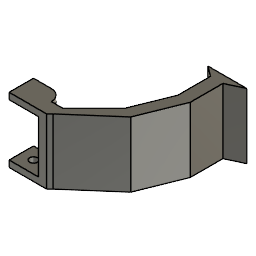
neck (Assembly) (Autodesk Fusion 360 archive; units mm, degrees)
design "tib 1"
Autodesk Fusion 360 part; units mm, degrees
note: some values were not read from the file. Chosen so that the rebuilt part matches the saved one: which face or edge a step refers to; which pieces of a blend or face edit are solid. Set by a fixed rule: which sketch regions a step uses.
sketch "Sketch1" plane through (0, 0, 0) normal (0, 0, 1) x (1, 0, 0)
  line L0 (0, 0) -> (50, 0)
  line L1 (50, 0) -> (50, 15)
  line L2 (50, 15) -> (0, 15)
  line L3 (0, 15) -> (0, 0)
  constraint horizontal L0
  constraint vertical L1
  constraint horizontal L2
  constraint vertical L3
  constraint coincident L0.start L3.end
extrude "Extrude1" add sketch "Sketch1" along normal blind 40
sketch "Sketch2" plane through (0, 0, 0) normal (-1, 0, 0) x (0, -1, 0)
  line L0 (-15, 0) -> (0, 0)
  line L1 (0, 0) -> (0, 40)
  line L2 (0, 40) -> (-15, 40)
  line L3 (-15, 40) -> (-15, 0)
  line L4 (2.957876, 2) -> (-22.207484, 2)
  line L5 (-22.207484, 2) -> (-22.207484, 38.000001)
  line L6 (-22.207484, 38.000001) -> (2.957876, 38.000001)
  line L7 (2.957876, 38.000001) -> (2.957876, 2)
  constraint horizontal L4
  constraint vertical L5
  constraint horizontal L6
  constraint vertical L7
extrude "Extrude2" cut sketch "Sketch2" against normal blind 46 contours L1 L3 L4 L6 picked at (-10, 26)
sketch "Sketch3" plane through (0, 0, 40) normal (0, 0, 1) x (-1, 0, 0)
  line L0 (0, -15) -> (0, 0)
  line L1 (0, 0) -> (-50, 0)
  line L2 (-50, 0) -> (-50, -15)
  line L3 (-50, -15) -> (0, -15)
  circle A0 centre (-7.5, -7.5) radius 2.4
  dimension "d5" = 4.8
  measures "d5" diameter of A0
extrude "Extrude3" cut sketch "Sketch3" against normal blind 50 contours A0 picked at (-7.452057, -6.860244)
sketch "Sketch4" plane through (0, 0, 0) normal (0, 0, -1) x (1, 0, 0)
  circle A0 centre (7.5, -7.5) radius 2.4
  line L0 (0, 0) -> (0, -15)
  line L1 (0, -15) -> (50, -15)
  line L2 (50, -15) -> (50, 0)
  line L3 (50, 0) -> (0, 0)
  circle A1 centre (7.5, -7.5) radius 4
  dimension "d8" = 8
  constraint concentric A0 A1
  measures "d8" diameter of A1
extrude "Extrude4" cut sketch "Sketch4" against normal blind 7 contours A1 picked at (10.951775, -7.698723)
extrude "Extrude5" add 1 faces at (46, 10, 26) along direction (-1, 0, 0) blind 30
extrude "Extrude6" cut 1 faces at (50, 5, 26.666667) along direction (-1, 0, 0) blind 25
chamfer "Chamfer1" distance 7 angle 45 1 edges at (25, 15, 20)
chamfer "Chamfer2" distance 2 angle 45 1 edges at (25, 0, 20)
extrude "Extrude7" add 1 faces at (22.666667, 10.333333, 13.333333) along direction (0.70710678, 0.70710678, 0) blind 30
chamfer "Chamfer3" distance 7 angle 45 1 edges at (39.213203, 36.213203, 20)
extrude "Extrude8" add 1 faces at (40.863119, 31.263456, 13.333333) along direction (0, 1, 0) blind 25
sketch "Sketch5" plane through (0, 0, 0) normal (0, 0, -1) x (1, 0, 0)
  circle A0 centre (7.5, -7.5) radius 4
  line L0 (44.162951, -31.263456) -> (46.213203, -29.213203)
  line L1 (46.213203, -29.213203) -> (25, -8)
  line L2 (25, -8) -> (25, -2)
  line L3 (25, -2) -> (23, 0)
  line L4 (23, 0) -> (0, 0)
  line L5 (0, 0) -> (0, -15)
  line L6 (0, -15) -> (18, -15)
  line L7 (18, -15) -> (34.263456, -31.263456)
  line L8 (34.263456, -31.263456) -> (34.263456, -56.263456)
  line L9 (34.263456, -56.263456) -> (44.162951, -56.263456)
  line L10 (44.162951, -56.263456) -> (44.162951, -31.263456)
  line L11 (44.162951, -31.263456) -> (44.162951, -27.162951)
  line L12 (44.162951, -27.162951) -> (46.213203, -29.213203)
  line L13 (44.162951, -31.263456) -> (46.213203, -29.213203)
  constraint parallel L10 L11
extrude "Extrude9" cut sketch "Sketch5" against normal blind 43 contours L0 L1 L11 L12 L13 picked at (44.846368, -29.213203)
chamfer "Chamfer4" distance 3 angle 45 1 edges at (44.162951, 56.263456, 20)
sketch "Sketch6" plane through (0, 0, 0) normal (0, 0, -1) x (1, 0, 0)
  line L0 (41.162951, -56.263456) -> (44.162951, -53.263456)
  line L1 (44.162951, -53.263456) -> (44.162951, -27.162951)
  line L2 (44.162951, -27.162951) -> (25, -8)
  line L3 (25, -8) -> (25, -2)
  line L4 (25, -2) -> (23, 0)
  line L5 (23, 0) -> (0, 0)
  line L6 (0, 0) -> (0, -15)
  line L7 (0, -15) -> (18, -15)
  line L8 (18, -15) -> (34.263456, -31.263456)
  line L9 (34.263456, -31.263456) -> (34.263456, -56.263456)
  line L10 (34.263456, -56.263456) -> (41.162951, -56.263456)
  circle A0 centre (7.5, -7.5) radius 4
  circle A1 centre (7.5, -7.5) radius 2.4
  dimension "d25" = 4.8
  constraint concentric A0 A1
  measures "d25" diameter of A1
extrude "Extrude10" add sketch "Sketch6" against normal blind 2 contours A0 picked at (10.951775, -7.698723)
sketch "Sketch7" plane through (0, 0, 38.000001) normal (0, 0, -1) x (1, 0, 0)
  line L0 (16, -15) -> (16, 0)
  line L1 (16, 0) -> (0, 0)
  line L2 (0, 0) -> (0, -15)
  line L3 (0, -15) -> (16, -15)
  circle A0 centre (7.5, -7.5) radius 2.4
  circle A1 centre (7.5, -7.5) radius 4
  dimension "d28" = 8
  constraint concentric A0 A1
  measures "d28" diameter of A1
extrude "Extrude11" cut sketch "Sketch7" against normal blind 3 contours A1 picked at (10.951775, -7.698723)
sketch "Sketch8" plane through (0, 0, 38.000001) normal (0, 0, -1) x (1, 0, 0)
  circle A0 centre (7.5, -7.5) radius 4
  line L0 (16, -15) -> (16, 0)
  line L1 (16, 0) -> (0, 0)
  line L2 (0, 0) -> (0, -15)
  line L3 (0, -15) -> (16, -15)
  circle A1 centre (7.5, -7.5) radius 4
  constraint concentric A0 A1
extrude "Extrude12" add sketch "Sketch8" along normal blind 2 and the other way blind 2 contours A0 A1 picked at (6.101654, -8.048811)
extrude "Extrude13" cut 1 faces at (36.563288, 56.263456, 26.666667) along direction (0, -1, 0) blind 25
sketch "Sketch9" plane through (0, 0, 40) normal (0, 0, 1) x (-1, 0, 0)
  line L0 (-41.162951, -56.263456) -> (-41.162951, -31.263456)
  line L1 (-41.162951, -31.263456) -> (-34.263456, -31.263456)
  line L2 (-34.263456, -31.263456) -> (-18, -15)
  line L3 (-18, -15) -> (0, -15)
  line L4 (0, -15) -> (0, 0)
  line L5 (0, 0) -> (-23, 0)
  line L6 (-23, 0) -> (-25, -2)
  line L7 (-25, -2) -> (-25, -8)
  line L8 (-25, -8) -> (-44.162951, -27.162951)
  line L9 (-44.162951, -27.162951) -> (-44.162951, -53.263456)
  line L10 (-44.162951, -53.263456) -> (-41.162951, -56.263456)
extrude "Extrude14" cut 1 faces at (41.162951, 47.930123, 13.333333) along direction (1, 0, 0) blind 26
sketch "Sketch10" plane through (0, 0, 40) normal (0, 0, 1) x (-1, 0, 0)
  line L0 (-44.000001, -27) -> (-34.000001, -31)
  line L1 (-34.000001, -31) -> (-34.243008, -31.24155)
  line L2 (-34.243008, -31.24155) -> (-44.199999, -31.24155)
  line L3 (-44.199999, -31.24155) -> (-44.199999, -27.099999)
  line L4 (-44.199999, -27.099999) -> (-44.000001, -27)
  constraint horizontal L2
  constraint perpendicular L2 L3
extrude "Extrude15" cut sketch "Sketch10" against normal blind 45
delete_face "DeleteFace1" 1 faces at (40.863119, 31.263456, 13.333333)
delete_face "DeleteFace2" 1 faces at (40.856303, 34.548684, 40)
extrude "Extrude16" add 2 faces at (40.666667, 28.333334, 36.161338) (40.666667, 28.333334, 18.989342) along direction (0.37139068, 0.92847669, 0) blind 40
chamfer "Chamfer5" distance 5 angle 45 1 edges at (58.855628, 64.139068, 20)
extrude "Extrude17" add 1 faces at (13.966667, 7.5, 2) along direction (0, 0, 1) blind 4
extrude "Extrude18" cut 1 faces at (46.618101, 52.878584, 0) along direction (0, 0, 1) blind 2
extrude "Extrude19" cut 1 faces at (16, 10, 16.666667) along direction (1, 0, 0) blind 2
sketch "Sketch11" plane through (0, 0, 40) normal (0, 0, 1) x (-1, 0, 0)
  line L0 (-56.998674, -59.496685) -> (-54.213244, -65.996021)
  line L1 (-54.213244, -65.996021) -> (-48.855628, -68.139068)
  line L2 (-48.855628, -68.139068) -> (-34.000001, -31)
  line L3 (-34.000001, -31) -> (-18, -15)
  line L4 (-18, -15) -> (0, -15)
  line L5 (0, -15) -> (0, 0)
  line L6 (0, 0) -> (-23, 0)
  line L7 (-23, 0) -> (-25, -2)
  line L8 (-25, -2) -> (-25, -8)
  line L9 (-25, -8) -> (-44.000001, -27)
  line L10 (-44.000001, -27) -> (-56.998674, -59.496685)
  line L11 (-56.998674, -59.496685) -> (-60.937867, -50.305234)
  line L12 (-60.937867, -50.305234) -> (-50.499337, -24.208909)
  line L13 (-50.499337, -24.208909) -> (-25, -2)
  line L14 (-18, -15) -> (-18, -8)
  line L15 (-18, -8) -> (-25, -8)
  dimension "d50" = 10
  constraint parallel L0 L11
  constraint parallel L10 L12
  constraint coincident L7.end L8.start
  constraint coincident L3.end L4.start
  constraint perpendicular L4 L14
  constraint coincident L8.end L9.start
extrude "Extrude20" add sketch "Sketch11" against normal blind 38 contours L8 L9 L10 L11 L12 L13 picked at (-53.978847, -45.60064)
extrude "Extrude21" cut sketch "Sketch11" against normal blind 40 contours L0 L1 L2 L3 L9 L10 L14 L15 picked at (-46.618101, -52.878584)
extrude "Extrude22" add sketch "Sketch11" along normal blind 2 contours L8 L9 L10 L11 L12 L13 | L4 L5 L6 L7 L8 L14 L15 picked at (-53.978847, -45.60064) picked at (-6, -7.666667)
fillet "Fillet1" radius 7 2 edges at (18, 15, 4) (18, 15, 40)
sketch "Sketch15" plane through (0, 0, 42) normal (0, 0, 1) x (-1, 0, 0)
  arc A0 (-18, -8) -> (-11, -15) centre (-11, -8) ccw
  line L0 (-11, -15) -> (0, -15)
  line L1 (0, -15) -> (0, 0)
  line L2 (0, 0) -> (-23, 0)
  line L3 (-23, 0) -> (-25, -2)
  line L4 (-25, -2) -> (-50.499337, -24.208909)
  line L5 (-50.499337, -24.208909) -> (-60.937867, -50.305234)
  line L6 (-60.937867, -50.305234) -> (-56.998674, -59.496685)
  line L7 (-56.998674, -59.496685) -> (-44.000001, -27)
  line L8 (-44.000001, -27) -> (-25, -8)
  line L9 (-25, -8) -> (-18, -8)
  line L10 (-60.937867, -50.305234) -> (-53.322094, -50.305234)
  line L11 (-53.322094, -50.305234) -> (-56.998674, -59.496685)
  line L12 (-61.161175, -50.305234) -> (-56.998674, -59.496685)
  line L13 (-61.161175, -50.305234) -> (-60.899999, -50.305234)
  constraint horizontal L10
  constraint parallel L10 L13
extrude "Extrude23" cut sketch "Sketch15" against normal blind 41 contours L6 L7 L10 L11 L13 picked at (-57.073589, -53.369051)
extrude "Extrude24" add 1 faces at (58.399276, 50.305234, 28.666667) along direction (0, 1, 0) blind 20
sketch "Sketch16" plane through (0, 0, 2) normal (0, 0, -1) x (1, 0, 0)
  circle A0 centre (7.5, -7.5) radius 2.4
  line L0 (60.937867, -50.305234) -> (50.499337, -24.208909)
  line L1 (50.499337, -24.208909) -> (25, -2)
  line L2 (25, -2) -> (23, 0)
  line L3 (23, 0) -> (0, 0)
  line L4 (0, 0) -> (0, -15)
  line L5 (0, -15) -> (11, -15)
  arc A1 (11, -15) -> (18, -8) centre (11, -8) ccw
  line L6 (18, -8) -> (25, -8)
  line L7 (25, -8) -> (44.000001, -27)
  line L8 (44.000001, -27) -> (53.322094, -50.305234)
  line L9 (53.322094, -50.305234) -> (53.322094, -70.305234)
  line L10 (53.322094, -70.305234) -> (60.937867, -70.305234)
  line L11 (60.937867, -70.305234) -> (60.937867, -50.305234)
  line L12 (71.000001, -75.000001) -> (60.937867, -70.305234)
  line L13 (53.322094, -70.305234) -> (47.000001, -75.000001)
  line L14 (47.000001, -75.000001) -> (71.000001, -75.000001)
  constraint perpendicular L9 L14
extrude "Extrude25" add sketch "Sketch16" against normal blind 40 contours L10 L12 L13 L14 picked at (59.645956, -73.435079)

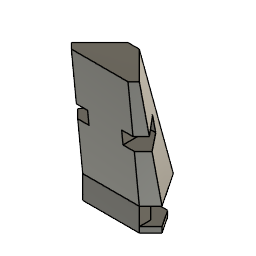
design "neck"
Autodesk Fusion 360 part; units mm, degrees
sketch "Sketch1" plane through (0, 0, 0) normal (0, 0, 1) x (1, 0, 0)
  line L0 (50, 30) -> (20, 30)
  line L1 (0, 0) -> (20, 30)
  line L2 (50, 30) -> (70, 0)
  line L3 (0, 0) -> (10, -10)
  line L4 (10, -10) -> (60, -10)
  line L5 (60, -10) -> (70, 0)
  constraint horizontal L0
  constraint coincident L1.start L3.start
  constraint perpendicular L3 L5
ref_plane "WorkPlane1" through (0, 0, 100) normal (0, 0, 1) x (1, 0, 0)
sketch "Sketch2" plane through (0, 0, 100) normal (0, 0, 1) x (1, 0, 0)
  line L0 (30, 10) -> (40, 10)
  line L1 (60, -20) -> (10, -20)
  line L2 (30, 10) -> (5, -15)
  line L3 (5, -15) -> (10, -20)
  line L4 (40, 10) -> (65, -15)
  line L5 (65, -15) -> (60, -20)
  constraint horizontal L0
  constraint horizontal L1
  constraint perpendicular L2 L3
  constraint parallel L3 L4
  constraint perpendicular L4 L5
loft "Loft1" add profiles "Sketch1", "Sketch2" section 1 section 2 makes body 1
ref_plane "WorkPlane2" through (35, 10, 50) normal (0, 0, -1) x (-1, 0, 0)
sketch "Sketch3" plane through (0, 0, 50) normal (0, 0, -1) x (-1, 0, 0)
  line L0 (0.4452, 9.35) -> (-20, 9.35)
  line L1 (-20, 9.35) -> (-20, -30.9261)
  line L2 (-20, -30.9261) -> (0.4452, -30.9261)
  line L3 (0.4452, -30.9261) -> (0.4452, 9.35)
  line L4 (-69.0117, 9.35) -> (-50, 9.35)
  line L5 (-50, 9.35) -> (-50, -30.2583)
  line L6 (-50, -30.2583) -> (-69.0117, -30.2583)
  line L7 (-69.0117, -30.2583) -> (-69.0117, 9.35)
  constraint horizontal L0
  constraint vertical L1
  constraint horizontal L2
  constraint vertical L3
  constraint horizontal L4
  constraint vertical L5
  constraint horizontal L6
  constraint vertical L7
extrude "Extrude1" cut sketch "Sketch3" along normal blind -6 and the other way blind -6 bodies 1
ref_plane "WorkPlane3" through (35, 10, -15.5) normal (0, 0, -1) x (-1, 0, 0)
sketch "Sketch4" plane through (0, 0, -15.5) normal (0, 0, -1) x (-1, 0, 0)
  line L0 (-70, 0) -> (-60, 15)
  line L1 (0, 0) -> (-10, -10)
  line L2 (-10, -10) -> (-60, -10)
  line L3 (-60, -10) -> (-70, 0)
  line L4 (-10, 15) -> (0, 0)
  line L5 (-60, 15) -> (-10, 15)
  constraint coincident L1.start L4.end
  constraint horizontal L5
extrude "Extrude2" add sketch "Sketch4" along normal blind 5 separate body makes body 2
sketch "Sketch5" plane through (0, 0, 0) normal (0, 0, -1) x (1, 0, 0)
  line L0 (10, 10) -> (0, 0)
  line L1 (0, 0) -> (20, -30)
  line L2 (20, -30) -> (50, -30)
  line L3 (50, -30) -> (70, 0)
  line L4 (70, 0) -> (60, 10)
  line L5 (60, 10) -> (10, 10)
  line L6 (10, 10) -> (60, 10)
  line L7 (60, 10) -> (60, 0)
  line L8 (60, 0) -> (10, 0)
  line L9 (10, 0) -> (10, 10)
  constraint horizontal L6
  constraint vertical L7
  constraint horizontal L8
  constraint vertical L9
  constraint coincident L0.start L5.end
extrude "Extrude3" add sketch "Sketch5" along normal blind 20 contours L5 L6 L7 L8 L9 bodies 1 2

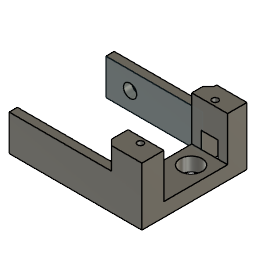
design "cosa"
Autodesk Fusion 360 part; units mm, degrees
sketch "Sketch1" plane through (0, 0, 0) normal (0, 0, 1) x (1, 0, 0)
  line L0 (6.5, -11.5) -> (-6.5, -11.5)
  line L1 (-6.5, -11.5) -> (-6.5, 11.5)
  line L2 (-6.5, 11.5) -> (6.5, 11.5)
  line L3 (6.5, 11.5) -> (6.5, -11.5)
  line L4 (6.5, -11.5) -> (-6.5, 11.5) construction
  line L5 (-6.5, -11.5) -> (6.5, 11.5) construction
  line L6 (6.5, -11.5) -> (-6.5, -11.5)
  line L7 (-6.5, -11.5) -> (-6.5, -17.5)
  line L8 (-6.5, -17.5) -> (6.5, -17.5)
  line L9 (6.5, -17.5) -> (6.5, -11.5)
  line L10 (6.5, 11.5) -> (-6.5, 11.5)
  line L11 (-6.5, 11.5) -> (-6.5, 17.5)
  line L12 (-6.5, 17.5) -> (6.5, 17.5)
  line L13 (6.5, 17.5) -> (6.5, 11.5)
  dimension "d1" = 13
  dimension "d2" = 23
  dimension "d3" = 6
  dimension "d4" = 6
  constraint horizontal L0
  constraint perpendicular L0 L1
  constraint parallel L0 L2
  constraint parallel L1 L3
  constraint coincident L4 origin
  constraint coincident L5 origin
  constraint horizontal L6
  constraint vertical L7
  constraint horizontal L8
  constraint vertical L9
  constraint horizontal L10
  constraint vertical L11
  constraint horizontal L12
  constraint vertical L13
  measures "d1" distance of L1.end L2.end
  measures "d2" distance of L0.end L1.end
  measures "d3" distance of L0.start L8.end
  measures "d4" distance of L2.end L12.end
extrude "Extrude1" add sketch "Sketch1" along normal blind 21 contours L0 L6 L7 L8 L9 | L2 L10 L11 L12 L13 makes body 1 at (-2.1667, -17.5, 7) makes body 2 at (-2.1667, 17.5, 7)
extrude "Extrude2" add sketch "Sketch1" along normal blind 5 contours L0 L1 L2 L3 L6 L10 bodies 1 2
sketch "Sketch2" plane through (0, 0, 5) normal (0, 0, 1) x (-1, 0, 0)
  line L0 (-6.5, 11.5) -> (-6.5, -11.5)
  line L1 (-6.5, -11.5) -> (6.5, -11.5)
  line L2 (6.5, -11.5) -> (6.5, 11.5)
  line L3 (6.5, 11.5) -> (-6.5, 11.5)
  circle A0 centre (0, -5.75) radius 4
  dimension "d9" = 8
  measures "d9" diameter of A0
extrude "Extrude3" cut sketch "Sketch2" against normal blind 6.5 contours A0 bodies 1
sketch "Sketch3" plane through (-6.5, 0, 0) normal (-1, 0, 0) x (0, -1, 0)
  line L0 (-17.5, 0) -> (17.5, 0)
  line L1 (17.5, 0) -> (17.5, 21)
  line L2 (17.5, 21) -> (11.5, 21)
  line L3 (11.5, 21) -> (11.5, 5)
  line L4 (11.5, 5) -> (-11.5, 5)
  line L5 (-11.5, 5) -> (-11.5, 21)
  line L6 (-11.5, 21) -> (-17.5, 21)
  line L7 (-17.5, 21) -> (-17.5, 0)
  line L8 (-17.5, 0) -> (-14.5, 0)
  line L9 (-14.5, 0) -> (-14.5, 13)
  line L10 (-14.5, 13) -> (-17.5, 13)
  line L11 (-17.5, 13) -> (-17.5, 0)
  line L12 (17.5, 0) -> (14.5, 0)
  line L13 (14.5, 0) -> (14.5, 13)
  line L14 (14.5, 13) -> (17.5, 13)
  line L15 (17.5, 13) -> (17.5, 0)
  dimension "d12" = 3
  constraint horizontal L8
  constraint vertical L9
  constraint horizontal L10
  constraint vertical L11
  constraint coincident L0.start L7.end
  constraint horizontal L12
  constraint vertical L13
  constraint horizontal L14
  constraint vertical L15
  constraint coincident L0.end L1.start
  measures "d12" distance of L0.end L12.end
extrude "Extrude4" add sketch "Sketch3" along normal blind 25 contours L0 L7 L8 L9 L10 L11 | L0 L1 L12 L13 L14 L15 bodies 1
chamfer "Chamfer1" distance 2 angle 45 2 edges at (-6.5, 17.5, 17) (-6.5, -17.5, 17) on bodies 1
sketch "Sketch4" plane through (0, -14.5, 0) normal (0, 1, 0) x (-1, 0, 0)
  line L0 (6.5, 13) -> (6.5, 0)
  line L1 (6.5, 0) -> (31.5, 0)
  line L2 (31.5, 0) -> (31.5, 13)
  line L3 (31.5, 13) -> (6.5, 13)
  circle A0 centre (25.25, 6.5) radius 4
  dimension "d16" = 8
  measures "d16" diameter of A0
extrude "Extrude5" add sketch "Sketch4" along normal blind 2 contours A0 bodies 1
sketch "Sketch5" plane through (0, 17.5, 0) normal (0, 1, 0) x (-1, 0, 0)
  line L0 (4.5, 13) -> (4.5, 21)
  line L1 (4.5, 21) -> (-6.5, 21)
  line L2 (-6.5, 21) -> (-6.5, 0)
  line L3 (-6.5, 0) -> (31.5, 0)
  line L4 (31.5, 0) -> (31.5, 13)
  line L5 (31.5, 13) -> (4.5, 13)
  line L6 (-3, -10) -> (3, -10)
  line L7 (3, -10) -> (3, 10)
  line L8 (3, 10) -> (-3, 10)
  line L9 (-3, 10) -> (-3, -10)
  line L10 (-3, -10) -> (3, 10) construction
  line L11 (3, -10) -> (-3, 10) construction
  constraint horizontal L6
  constraint perpendicular L6 L7
  constraint parallel L6 L8
  constraint parallel L7 L9
  constraint coincident L10 origin
  constraint coincident L11 origin
extrude "Extrude6" cut sketch "Sketch5" against normal blind 6 contours L3 L7 L8 L9 bodies 1
extrude "Extrude7" add 2 faces at (-31.5, 16.5, 8.6667) (-31.5, -15.5, 8.6667) along direction (-1, 0, 0) blind 10 on bodies 1 bodies 1
extrude "Extrude8" cut 1 faces at (-26.4956, -12.5, 5.7272) along direction (0, -1, 0) blind 2 on bodies 1 bodies 1
extrude "Extrude9" add 1 faces at (-13.1667, -17.5, 4.3333) along direction (0, -1, 0) blind 5 on bodies 1 bodies 1
extrude "Extrude10" cut 1 faces at (-18.1667, -14.5, 4.3333) along direction (0, -1, 0) blind 2 on bodies 1 bodies 1
extrude "Extrude11" cut 1 faces at (-13.1667, -22.5, 4.3333) along direction (0, 1, 0) blind 3 on bodies 1 bodies 1
sketch "Sketch6" plane through (0, -16.5, 0) normal (0, 1, 0) x (-1, 0, 0)
  line L0 (6.5, 13) -> (6.5, 0)
  line L1 (6.5, 0) -> (41.5, 0)
  line L2 (41.5, 0) -> (41.5, 13)
  line L3 (41.5, 13) -> (6.5, 13)
  line L4 (24, 13) -> (24, 0)
  circle A0 centre (32.75, 6.5) radius 4
  dimension "d31" = 8
  constraint midpoint L3 L4.start
  constraint midpoint L1 L4.end
  measures "d31" diameter of A0
extrude "Extrude12" add sketch "Sketch6" along normal blind 2 contours A0 bodies 1
sketch "Sketch7" plane through (0, 0, 13) normal (0, 0, 1) x (-1, 0, 0)
  line L0 (41.5, 19.5) -> (4.5, 19.5)
  line L1 (4.5, 19.5) -> (4.5, 17.5)
  line L2 (4.5, 17.5) -> (6.5, 15.5)
  line L3 (6.5, 15.5) -> (6.5, 16.5)
  line L4 (6.5, 16.5) -> (41.5, 16.5)
  line L5 (41.5, 16.5) -> (41.5, 19.5)
  line L6 (6.5, 19.5) -> (6.5, 15.5)
  line L7 (6.5, 19.5) -> (4.5, 19.5)
  constraint coincident L0 L6.start
  constraint coincident L2.end L3.start
  constraint coincident L0.end L1.start
extrude "Extrude13" add 1 faces at (-4.5, -18.1667, 15.6667) along direction (-1, 0, 0) blind 2 on bodies 1 bodies 1
extrude "Extrude14" add 1 faces at (-5.8333, -17.5, 15.6667) along direction (0, 1, 0) blind 2 on bodies 1 bodies 1
chamfer "Chamfer2" distance 2 angle 45 1 edges at (-6.5, -19.5, 17) on bodies 1
extrude "Extrude15" cut 1 faces at (-18.1667, 14.5, 4.3333) along direction (0, 1, 0) blind 1 on bodies 1 bodies 1
extrude "Extrude16" add 1 faces at (-16.3333, 17.5, 4.3333) along direction (0, 1, 0) blind 1 on bodies 1 bodies 1
sketch "Sketch8" plane through (0, 15.5, 0) normal (0, -1, 0) x (1, 0, 0)
  line L0 (-6.5, 0) -> (-6.5, 13)
  line L1 (-6.5, 13) -> (-41.5, 13)
  line L2 (-41.5, 13) -> (-41.5, 0)
  line L3 (-41.5, 0) -> (-6.5, 0)
extrude "Extrude17" cut 1 faces at (-31.963, -14.5, 4.8658) along direction (0, 1, 0) blind 38 on bodies 1 bodies 1
sketch "Sketch9" plane through (0, 18.5, 0) normal (0, 1, 0) x (-1, 0, 0)
  circle A0 centre (32.75, 6.5) radius 4
  line L0 (-3, 0) -> (-3, 10)
  line L1 (-3, 10) -> (3, 10)
  line L2 (3, 10) -> (3, 0)
  line L3 (3, 0) -> (41.5, 0)
  line L4 (41.5, 0) -> (41.5, 13)
  line L5 (41.5, 13) -> (4.5, 13)
  line L6 (4.5, 13) -> (4.5, 21)
  line L7 (4.5, 21) -> (-6.5, 21)
  line L8 (-6.5, 21) -> (-6.5, 0)
  line L9 (-6.5, 0) -> (-3, 0)
  circle A1 centre (32.75, 6.5) radius 1.25
  dimension "d45" = 2.5
  constraint concentric A0 A1
  measures "d45" diameter of A1
extrude "Extrude18" add sketch "Sketch9" against normal blind 3 contours A0 bodies 1
extrude "Extrude19" cut 1 faces at (-1, 16.1667, 10) along direction (0, 0, 1) blind 1 on bodies 1 bodies 1
sketch "Sketch10" plane through (0, 0, 21) normal (0, 0, 1) x (-1, 0, 0)
  line L0 (4.5, -17.5) -> (6.5, -15.5)
  line L1 (6.5, -15.5) -> (6.5, -11.5)
  line L2 (6.5, -11.5) -> (-6.5, -11.5)
  line L3 (-6.5, -11.5) -> (-6.5, -18.5)
  line L4 (-6.5, -18.5) -> (4.5, -18.5)
  line L5 (4.5, -18.5) -> (4.5, -17.5)
  circle A0 centre (0, -13.5) radius 1.1
  dimension "d51" = 2.2
  measures "d51" diameter of A0
extrude "Extrude20" cut sketch "Sketch10" against normal blind 4 contours A0 bodies 1
sketch "Sketch11" plane through (0, 0, 21) normal (0, 0, 1) x (-1, 0, 0)
  line L0 (6.5, 17.5) -> (4.5, 19.5)
  line L1 (4.5, 19.5) -> (-6.5, 19.5)
  line L2 (-6.5, 19.5) -> (-6.5, 11.5)
  line L3 (-6.5, 11.5) -> (6.5, 11.5)
  line L4 (6.5, 11.5) -> (6.5, 17.5)
  circle A0 centre (0, 13.5) radius 1.1
  dimension "d55" = 2.2
  measures "d55" diameter of A0
extrude "Extrude21" cut sketch "Sketch11" against normal blind 4 contours A0 bodies 1
sketch "Sketch12" plane through (0, 18.5, 0) normal (0, 1, 0) x (-1, 0, 0)
  line L0 (-3, 0) -> (-3, 11)
  line L1 (-3, 11) -> (3, 11)
  line L2 (3, 11) -> (3, 0)
  line L3 (3, 0) -> (41.5, 0)
  line L4 (41.5, 0) -> (41.5, 13)
  line L5 (41.5, 13) -> (4.5, 13)
  line L6 (4.5, 13) -> (4.5, 21)
  line L7 (4.5, 21) -> (-6.5, 21)
  line L8 (-6.5, 21) -> (-6.5, 0)
  line L9 (-6.5, 0) -> (-3, 0)
  circle A0 centre (32.75, 6.5) radius 1.25
  circle A1 centre (32.75, 6.5) radius 2.4
  dimension "d58" = 4.8
  constraint concentric A0 A1
  measures "d58" diameter of A1
extrude "Extrude22" cut sketch "Sketch12" against normal blind 4.5 contours A1 bodies 1
sketch "Sketch13" plane through (0, 0, 0) normal (0, 0, -1) x (1, 0, 0)
  circle A0 centre (0, -5.75) radius 4
  line L0 (-6.5, 16.5) -> (-6.5, -15.5)
  line L1 (-6.5, -15.5) -> (-41.5, -15.5)
  line L2 (-41.5, -15.5) -> (-41.5, -18.5)
  line L3 (-41.5, -18.5) -> (-3, -18.5)
  line L4 (-3, -18.5) -> (-3, -11.5)
  line L5 (-3, -11.5) -> (3, -11.5)
  line L6 (3, -11.5) -> (3, -18.5)
  line L7 (3, -18.5) -> (6.5, -18.5)
  line L8 (6.5, -18.5) -> (6.5, 19.5)
  line L9 (6.5, 19.5) -> (-41.5, 19.5)
  line L10 (-41.5, 19.5) -> (-41.5, 16.5)
  line L11 (-41.5, 16.5) -> (-6.5, 16.5)
  line L12 (6.5, -11.5) -> (-6.5, -11.5)
  line L13 (-6.5, -11.5) -> (-6.5, 1)
  line L14 (6.5, 1) -> (-6.5, 1)
  line L15 (6.5, 1) -> (6.5, -11.5)
  constraint coincident L8 L12.start
  constraint coincident L0 L12.end
  constraint perpendicular L0 L12
  constraint coincident L0 L13.end
  constraint coincident L8 L14.start
  constraint perpendicular L13 L14
extrude "Extrude23" add sketch "Sketch13" against normal blind 5 contours A0 bodies 1
sketch "Sketch14" plane through (0, 0, 0) normal (0, 0, -1) x (1, 0, 0)
  line L0 (-6.5, 16.5) -> (-6.5, -15.5)
  line L1 (-6.5, -15.5) -> (-41.5, -15.5)
  line L2 (-41.5, -15.5) -> (-41.5, -18.5)
  line L3 (-41.5, -18.5) -> (-3, -18.5)
  line L4 (-3, -18.5) -> (-3, -11.5)
  line L5 (-3, -11.5) -> (3, -11.5)
  line L6 (3, -11.5) -> (3, -18.5)
  line L7 (3, -18.5) -> (6.5, -18.5)
  line L8 (6.5, -18.5) -> (6.5, 19.5)
  line L9 (6.5, 19.5) -> (-41.5, 19.5)
  line L10 (-41.5, 19.5) -> (-41.5, 16.5)
  line L11 (-41.5, 16.5) -> (-6.5, 16.5)
  circle A0 centre (0, -4.8) radius 4
  dimension "d67" = 8
  measures "d67" diameter of A0
extrude "Extrude24" cut sketch "Sketch14" against normal blind 5 contours A0 bodies 1
